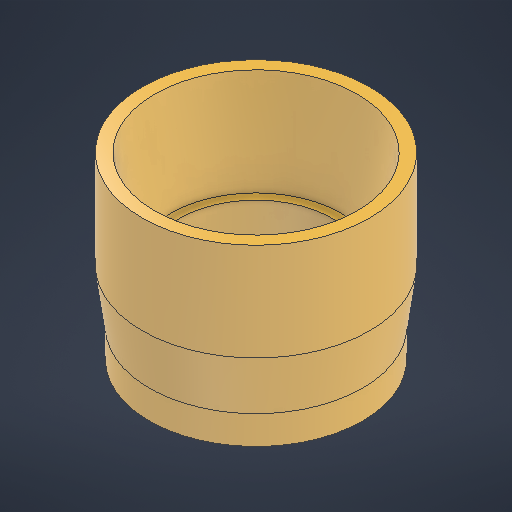
# Autodesk Inventor part: PARTE_INTERIOR_FENOLICO_TOBERA
Saved by Autodesk Inventor 2025 (Build 290162010, 162A)
## iProperties
Created: 2024-07-24
Part Number: PARTE_INTERIOR_FENOLICO_TOBERA
Material: Resina fenólica
Document SubType Name: Modeling
Designer: hansm
Mass: 74.866 g
Surface Area: 197.34 cm^2
Volume: 54.2507 cm^3
Density: 1.38 g/cm^3
Appearance: Abedul - Natural pulido
Author: hansm
Autodesk Inventor part; units mm, degrees
ref_plane "YZ Plane" through (0, 0, 0) normal (1, 0, 0) x (0, 1, 0)
ref_plane "XZ Plane" through (0, 0, 0) normal (0, 1, 0) x (-1, 0, 0)
ref_plane "XY Plane" through (0, 0, 0) normal (0, 0, 1) x (1, 0, 0)
sketch "Boceto1" plane through (0, 0, 0) normal (0, 0, 1) x (1, 0, 0)
  line L0 (-32, 50.5) -> (-32, 23)
  line L1 (-32, 23) -> (-30, 8)
  line L2 (-30, 8) -> (-30, 0)
  line L3 (-32, 50.5) -> (-28.5, 50.5)
  line L4 (-24, 23.6746) -> (-21.5, 23.6746)
  line L5 (-21.5, 23.6746) -> (-27, 0)
  line L6 (-27, 0) -> (-30, 0)
  line L7 (-28.5, 50.5) -> (-24, 23.6746)
  line L8 (0, -10.1) -> (0, 60.6) projected
  point P0 (0, 0)
  point P1 (0, 0)
  dimension "d2" = 2
  dimension "d3" = 8
  dimension "d4" = 15
  dimension "d14" = 3.5
  dimension "d15" = 3
  dimension "d16" = 2.5
  dimension "d17" = 4.5
  constraints: 16 end point, 2 horizontal, 2 parallel, 1 vertical
  measures "d2" horizontal distance of L2.end L0.end
  measures "d3" distance of L1.end L2.end
  measures "d4" vertical distance of L1.end L0.end
  measures "d14" distance of L0.start L3.end
  measures "d15" distance of L5.end L2.end
  measures "d16" distance of L4.start L4.end
  measures "d17" horizontal distance of L4.start L3.end
revolve "Revolución1" add sketch "Boceto1" angle 360 about axis through (0, -10, 0) along (0, 1, 0)
